Autodesk Fusion 360 part; units mm, degrees
note: some values were not read from the file. Set by a fixed rule: which sketch regions a step uses.
(part 16 of 59)
  spline S89 degree 5 poles (30.8773, 9.745) (30.8749, 9.7461) (30.87, 9.7485) (30.8627, 9.752) (30.853, 9.7566) (30.8408, 9.7624) (30.8287, 9.7681) (30.8165, 9.7738) (30.8044, 9.7795) (30.7924, 9.7851) (30.7803, 9.7908) (30.7683, 9.7964) (30.7563, 9.8019) (30.7443, 9.8075) (30.7323, 9.813) (30.7204, 9.8185) (30.7085, 9.8239) (30.6966, 9.8293) (30.6847, 9.8347) (30.6728, 9.8401) (30.661, 9.8455) (30.6492, 9.8508) (30.6374, 9.8561) (30.6256, 9.8613) (30.6139, 9.8665) (30.6022, 9.8717) (30.5905, 9.8769) (30.5788, 9.8821) (30.5672, 9.8872) (30.5555, 9.8923) (30.5439, 9.8973) (30.5324, 9.9023) (30.5208, 9.9073) (30.5093, 9.9123) (30.4978, 9.9173) (30.4863, 9.9222) (30.4749, 9.9271) (30.4634, 9.9319) (30.452, 9.9368) (30.4407, 9.9416) (30.4293, 9.9463) (30.418, 9.9511) (30.4067, 9.9558) (30.3954, 9.9605) (30.3841, 9.9652) (30.3729, 9.9698) (30.3617, 9.9744) (30.3506, 9.979) (30.3394, 9.9835) (30.3283, 9.9881) (30.3172, 9.9926) (30.3061, 9.997) (30.2951, 10.0015) (30.2841, 10.0059) (30.2731, 10.0103) (30.2621, 10.0146) (30.2512, 10.019) (30.2403, 10.0233) (30.2294, 10.0275) (30.2186, 10.0318) (30.2078, 10.036) (30.197, 10.0402) (30.1862, 10.0443) (30.1755, 10.0485) (30.1648, 10.0526) (30.1541, 10.0567) (30.1435, 10.0607) (30.1329, 10.0647) (30.1223, 10.0687) (30.1118, 10.0727) (30.1012, 10.0766) (30.0907, 10.0806) (30.0803, 10.0844) (30.0699, 10.0883) (30.0595, 10.0921) (30.0491, 10.0959) (30.0388, 10.0997) (30.0284, 10.1035) (30.0182, 10.1072) (30.0079, 10.1109) (29.9977, 10.1145) (29.9875, 10.1182) (29.9774, 10.1218) (29.9673, 10.1254) (29.9572, 10.1289) (29.9471, 10.1325) (29.9371, 10.136) (29.9271, 10.1394) (29.9172, 10.1429) (29.9073, 10.1463) (29.8974, 10.1497) (29.8875, 10.1531) (29.8777, 10.1564) (29.868, 10.1597) (29.8582, 10.163) (29.8485, 10.1663) (29.8388, 10.1695) (29.8292, 10.1727) (29.8196, 10.1759) (29.81, 10.179) (29.8005, 10.1822) (29.791, 10.1853) (29.7815, 10.1883) (29.7721, 10.1914) (29.7627, 10.1944) (29.7534, 10.1974) (29.7441, 10.2004) (29.7348, 10.2033) (29.7255, 10.2062) (29.7163, 10.2091) (29.7072, 10.212) (29.6981, 10.2148) (29.689, 10.2176) (29.6799, 10.2204) (29.6709, 10.2231) (29.6619, 10.2259) (29.653, 10.2286) (29.6441, 10.2312) (29.6353, 10.2339) (29.6265, 10.2365) (29.6177, 10.2391) (29.609, 10.2417) (29.6003, 10.2442) (29.5917, 10.2467) (29.583, 10.2492) (29.5745, 10.2517) (29.566, 10.2542) (29.5575, 10.2566) (29.5491, 10.259) (29.5407, 10.2613) (29.5323, 10.2637) (29.524, 10.266) (29.5158, 10.2683) (29.5075, 10.2705) (29.4994, 10.2728) (29.4912, 10.275) (29.4832, 10.2772) (29.4751, 10.2793) (29.4671, 10.2815) (29.4592, 10.2836) (29.4513, 10.2857) (29.4434, 10.2877) (29.4356, 10.2898) (29.4279, 10.2918) (29.4202, 10.2938) (29.4125, 10.2957) (29.4049, 10.2977) (29.3973, 10.2996) (29.3898, 10.3015) (29.3823, 10.3033) (29.3749, 10.3052) (29.3675, 10.307) (29.3602, 10.3088) (29.3529, 10.3105) (29.3457, 10.3123) (29.3386, 10.314) (29.3314, 10.3157) (29.3244, 10.3173) (29.3174, 10.319) (29.3104, 10.3206) (29.3035, 10.3222) (29.2967, 10.3238) (29.2899, 10.3253) (29.2831, 10.3269) (29.2764, 10.3284) (29.2698, 10.3298) (29.2632, 10.3313) (29.2567, 10.3327) (29.2502, 10.3341) (29.2438, 10.3355) (29.2374, 10.3369) (29.2311, 10.3382) (29.2249, 10.3395) (29.2187, 10.3408) (29.2126, 10.3421) (29.2065, 10.3433) (29.2005, 10.3446) (29.1946, 10.3458) (29.1887, 10.347) (29.1829, 10.3481) (29.1771, 10.3493) (29.1714, 10.3504) (29.1658, 10.3515) (29.1602, 10.3525) (29.1547, 10.3536) (29.1493, 10.3546) (29.1439, 10.3556) (29.1386, 10.3566) (29.1334, 10.3576) (29.1282, 10.3585) (29.1231, 10.3594) (29.118, 10.3603) (29.1131, 10.3612) (29.1081, 10.362) (29.1033, 10.3629) (29.0985, 10.3637) (29.0938, 10.3645) (29.0892, 10.3653) (29.0847, 10.366) (29.0802, 10.3668) (29.0758, 10.3675) (29.0714, 10.3682) (29.0672, 10.3688) (29.063, 10.3695) (29.0589, 10.3701) (29.0549, 10.3708) (29.0509, 10.3714) (29.047, 10.3719) (29.0432, 10.3725) (29.0395, 10.373) (29.0359, 10.3736) (29.0323, 10.3741) (29.0289, 10.3746) (29.0255, 10.375) (29.0222, 10.3755) (29.0189, 10.3759) (29.0158, 10.3763) (29.0128, 10.3767) (29.0098, 10.3771) (29.0069, 10.3775) (29.0041, 10.3778) (29.0015, 10.3781) (28.9989, 10.3785) (28.9963, 10.3788) (28.9939, 10.379) (28.9916, 10.3793) (28.9894, 10.3796) (28.9873, 10.3798) (28.9852, 10.38) (28.9833, 10.3802) (28.9815, 10.3804) (28.9798, 10.3806) (28.9781, 10.3808) (28.9766, 10.3809) (28.9752, 10.3811) (28.9739, 10.3812) (28.9727, 10.3813) (28.9716, 10.3814) (28.9706, 10.3815) (28.9698, 10.3816) (28.969, 10.3816) (28.9685, 10.3817) (28.9682, 10.3817) (28.968, 10.3817) (28.9679, 10.3817) knots -1 -1 -1 -1 -1 -1 -0.99583333 -0.99166667 -0.9875 -0.98333333 -0.97916667 -0.975 -0.97083333 -0.96666667 -0.9625 -0.95833333 -0.95416667 -0.95 -0.94583333 -0.94166667 -0.9375 -0.93333333 -0.92916667 -0.925 -0.92083333 -0.91666667 -0.9125 -0.90833333 -0.90416667 -0.9 -0.89583333 -0.89166667 -0.8875 -0.88333333 -0.87916667 -0.875 -0.87083333 -0.86666667 -0.8625 -0.85833333 -0.85416667 -0.85 -0.84583333 -0.84166667 -0.8375 -0.83333333 -0.82916667 -0.825 -0.82083333 -0.81666667 -0.8125 -0.80833333 -0.80416667 -0.8 -0.79583333 -0.79166667 -0.7875 -0.78333333 -0.77916667 -0.775 -0.77083333 -0.76666667 -0.7625 -0.75833333 -0.75416667 -0.75 -0.74583333 -0.74166667 -0.7375 -0.73333333 -0.72916667 -0.725 -0.72083333 -0.71666667 -0.7125 -0.70833333 -0.70416667 -0.7 -0.69583333 -0.69166667 -0.6875 -0.68333333 -0.67916667 -0.675 -0.67083333 -0.66666667 -0.6625 -0.65833333 -0.65416667 -0.65 -0.64583333 -0.64166667 -0.6375 -0.63333333 -0.62916667 -0.625 -0.62083333 -0.61666667 -0.6125 -0.60833333 -0.60416667 -0.6 -0.59583333 -0.59166667 -0.5875 -0.58333333 -0.57916667 -0.575 -0.57083333 -0.56666667 -0.5625 -0.55833333 -0.55416667 -0.55 -0.54583333 -0.54166667 -0.5375 -0.53333333 -0.52916667 -0.525 -0.52083333 -0.51666667 -0.5125 -0.50833333 -0.50416667 -0.5 -0.49583333 -0.49166667 -0.4875 -0.48333333 -0.47916667 -0.475 -0.47083333 -0.46666667 -0.4625 -0.45833333 -0.45416667 -0.45 -0.44583333 -0.44166667 -0.4375 -0.43333333 -0.42916667 -0.425 -0.42083333 -0.41666667 -0.4125 -0.40833333 -0.40416667 -0.4 -0.39583333 -0.39166667 -0.3875 -0.38333333 -0.37916667 -0.375 -0.37083333 -0.36666667 -0.3625 -0.35833333 -0.35416667 -0.35 -0.34583333 -0.34166667 -0.3375 -0.33333333 -0.32916667 -0.325 -0.32083333 -0.31666667 -0.3125 -0.30833333 -0.30416667 -0.3 -0.29583333 -0.29166667 -0.2875 -0.28333333 -0.27916667 -0.275 -0.27083333 -0.26666667 -0.2625 -0.25833333 -0.25416667 -0.25 -0.24583333 -0.24166667 -0.2375 -0.23333333 -0.22916667 -0.225 -0.22083333 -0.21666667 -0.2125 -0.20833333 -0.20416667 -0.2 -0.19583333 -0.19166667 -0.1875 -0.18333333 -0.17916667 -0.175 -0.17083333 -0.16666667 -0.1625 -0.15833333 -0.15416667 -0.15 -0.14583333 -0.14166667 -0.1375 -0.13333333 -0.12916667 -0.125 -0.12083333 -0.11666667 -0.1125 -0.10833333 -0.10416667 -0.1 -0.09583333 -0.09166667 -0.0875 -0.08333333 -0.07916667 -0.075 -0.07083333 -0.06666667 -0.0625 -0.05833333 -0.05416667 -0.05 -0.04583333 -0.04166667 -0.0375 -0.03333333 -0.02916667 -0.025 -0.02083333 -0.01666667 -0.0125 -0.00833333 -0.00416667 0 0 0 0 0 0
  spline S90 degree 5 poles (27.3251, 2.6528) (27.3252, 2.6528) (27.3254, 2.6527) (27.3257, 2.6526) (27.3262, 2.6525) (27.3269, 2.6522) (27.3277, 2.6519) (27.3286, 2.6516) (27.3296, 2.6513) (27.3308, 2.6509) (27.332, 2.6505) (27.3334, 2.65) (27.3348, 2.6495) (27.3364, 2.649) (27.338, 2.6485) (27.3398, 2.6479) (27.3416, 2.6473) (27.3435, 2.6467) (27.3456, 2.6461) (27.3477, 2.6454) (27.3499, 2.6447) (27.3523, 2.644) (27.3547, 2.6432) (27.3572, 2.6425) (27.3598, 2.6417) (27.3625, 2.6409) (27.3652, 2.64) (27.3681, 2.6392) (27.371, 2.6383) (27.3741, 2.6374) (27.3772, 2.6365) (27.3804, 2.6355) (27.3837, 2.6346) (27.387, 2.6336) (27.3905, 2.6326) (27.394, 2.6316) (27.3976, 2.6306) (27.4013, 2.6296) (27.4051, 2.6285) (27.409, 2.6275) (27.4129, 2.6264) (27.4169, 2.6253) (27.421, 2.6242) (27.4252, 2.6231) (27.4294, 2.622) (27.4337, 2.6208) (27.4381, 2.6197) (27.4426, 2.6185) (27.4471, 2.6173) (27.4517, 2.6162) (27.4564, 2.615) (27.4612, 2.6138) (27.466, 2.6126) (27.4709, 2.6113) (27.4759, 2.6101) (27.481, 2.6089) (27.4861, 2.6076) (27.4912, 2.6064) (27.4965, 2.6051) (27.5018, 2.6038) (27.5072, 2.6026) (27.5127, 2.6013) (27.5182, 2.6) (27.5238, 2.5987) (27.5294, 2.5974) (27.5352, 2.5961) (27.5409, 2.5948) (27.5468, 2.5935) (27.5527, 2.5921) (27.5587, 2.5908) (27.5647, 2.5895) (27.5709, 2.5882) (27.577, 2.5868) (27.5833, 2.5855) (27.5896, 2.5842) (27.5959, 2.5828) (27.6023, 2.5815) (27.6088, 2.5801) (27.6154, 2.5788) (27.622, 2.5775) (27.6286, 2.5761) (27.6353, 2.5748) (27.6421, 2.5734) (27.649, 2.5721) (27.6559, 2.5707) (27.6628, 2.5694) (27.6698, 2.568) (27.6769, 2.5667) (27.6841, 2.5653) (27.6912, 2.564) (27.6985, 2.5626) (27.7058, 2.5613) (27.7132, 2.5599) (27.7206, 2.5586) (27.728, 2.5572) (27.7356, 2.5559) (27.7431, 2.5546) (27.7508, 2.5532) (27.7585, 2.5519) (27.7662, 2.5506) (27.774, 2.5492) (27.7819, 2.5479) (27.7898, 2.5466) (27.7977, 2.5453) (27.8057, 2.544) (27.8138, 2.5427) (27.8219, 2.5414) (27.8301, 2.5401) (27.8383, 2.5388) (27.8466, 2.5375) (27.8549, 2.5362) (27.8633, 2.5349) (27.8717, 2.5336) (27.8802, 2.5324) (27.8887, 2.5311) (27.8973, 2.5299) (27.9059, 2.5286) (27.9146, 2.5274) (27.9233, 2.5261) (27.9321, 2.5249) (27.9409, 2.5237) (27.9498, 2.5224) (27.9587, 2.5212) (27.9677, 2.52) (27.9767, 2.5188) (27.9858, 2.5176) (27.9949, 2.5164) (28.004, 2.5153) (28.0133, 2.5141) (28.0225, 2.5129) (28.0318, 2.5118) (28.0412, 2.5106) (28.0506, 2.5095) (28.06, 2.5084) (28.0695, 2.5072) (28.079, 2.5061) (28.0886, 2.505) (28.0982, 2.5039) (28.1079, 2.5028) (28.1176, 2.5017) (28.1274, 2.5007) (28.1372, 2.4996) (28.147, 2.4986) (28.1569, 2.4975) (28.1668, 2.4965) (28.1768, 2.4955) (28.1868, 2.4945) (28.1969, 2.4935) (28.207, 2.4925) (28.2172, 2.4915) (28.2274, 2.4905) (28.2376, 2.4896) (28.2479, 2.4886) (28.2582, 2.4877) (28.2686, 2.4867) (28.279, 2.4858) (28.2894, 2.4849) (28.2999, 2.484) (28.3105, 2.4831) (28.321, 2.4823) (28.3317, 2.4814) (28.3423, 2.4805) (28.353, 2.4797) (28.3638, 2.4789) (28.3745, 2.4781) (28.3854, 2.4773) (28.3962, 2.4765) (28.4071, 2.4757) (28.4181, 2.4749) (28.429, 2.4742) (28.44, 2.4734) (28.4511, 2.4727) (28.4622, 2.472) (28.4733, 2.4713) (28.4845, 2.4706) (28.4957, 2.4699) (28.507, 2.4692) (28.5183, 2.4686) (28.5296, 2.4679) (28.541, 2.4673) (28.5524, 2.4667) (28.5638, 2.4661) (28.5753, 2.4655) (28.5868, 2.4649) (28.5984, 2.4644) (28.61, 2.4638) (28.6216, 2.4633) (28.6333, 2.4628) (28.645, 2.4623) (28.6567, 2.4618) (28.6685, 2.4613) (28.6803, 2.4608) (28.6922, 2.4604) (28.7041, 2.46) (28.716, 2.4595) (28.728, 2.4591) (28.74, 2.4588) (28.752, 2.4584) (28.7641, 2.458) (28.7762, 2.4577) (28.7883, 2.4573) (28.8005, 2.457) (28.8127, 2.4567) (28.8249, 2.4564) (28.8372, 2.4562) (28.8495, 2.4559) (28.8619, 2.4557) (28.8743, 2.4555) (28.8867, 2.4552) (28.8991, 2.4551) (28.9116, 2.4549) (28.9241, 2.4547) (28.9367, 2.4546) (28.9493, 2.4544) (28.9619, 2.4543) (28.9745, 2.4542) (28.9872, 2.4542) (29, 2.4541) (29.0127, 2.454) (29.0255, 2.454) (29.0383, 2.454) (29.0512, 2.454) (29.0641, 2.454) (29.077, 2.454) (29.0899, 2.4541) (29.1029, 2.4542) (29.1159, 2.4542) (29.129, 2.4543) (29.142, 2.4545) (29.1551, 2.4546) (29.1683, 2.4547) (29.1815, 2.4549) (29.1947, 2.4551) (29.2079, 2.4553) (29.2212, 2.4555) (29.2345, 2.4558) (29.2478, 2.456) (29.2612, 2.4563) (29.2745, 2.4566) (29.288, 2.4569) (29.3014, 2.4572) (29.3122, 2.4575) (29.3203, 2.4577) (29.3257, 2.4578) (29.3284, 2.4579) knots 0 0 0 0 0 0 0.00416667 0.00833333 0.0125 0.01666667 0.02083333 0.025 0.02916667 0.03333333 0.0375 0.04166667 0.04583333 0.05 0.05416667 0.05833333 0.0625 0.06666667 0.07083333 0.075 0.07916667 0.08333333 0.0875 0.09166667 0.09583333 0.1 0.10416667 0.10833333 0.1125 0.11666667 0.12083333 0.125 0.12916667 0.13333333 0.1375 0.14166667 0.14583333 0.15 0.15416667 0.15833333 0.1625 0.16666667 0.17083333 0.175 0.17916667 0.18333333 0.1875 0.19166667 0.19583333 0.2 0.20416667 0.20833333 0.2125 0.21666667 0.22083333 0.225 0.22916667 0.23333333 0.2375 0.24166667 0.24583333 0.25 0.25416667 0.25833333 0.2625 0.26666667 0.27083333 0.275 0.27916667 0.28333333 0.2875 0.29166667 0.29583333 0.3 0.30416667 0.30833333 0.3125 0.31666667 0.32083333 0.325 0.32916667 0.33333333 0.3375 0.34166667 0.34583333 0.35 0.35416667 0.35833333 0.3625 0.36666667 0.37083333 0.375 0.37916667 0.38333333 0.3875 0.39166667 0.39583333 0.4 0.40416667 0.40833333 0.4125 0.41666667 0.42083333 0.425 0.42916667 0.43333333 0.4375 0.44166667 0.44583333 0.45 0.45416667 0.45833333 0.4625 0.46666667 0.47083333 0.475 0.47916667 0.48333333 0.4875 0.49166667 0.49583333 0.5 0.50416667 0.50833333 0.5125 0.51666667 0.52083333 0.525 0.52916667 0.53333333 0.5375 0.54166667 0.54583333 0.55 0.55416667 0.55833333 0.5625 0.56666667 0.57083333 0.575 0.57916667 0.58333333 0.5875 0.59166667 0.59583333 0.6 0.60416667 0.60833333 0.6125 0.61666667 0.62083333 0.625 0.62916667 0.63333333 0.6375 0.64166667 0.64583333 0.65 0.65416667 0.65833333 0.6625 0.66666667 0.67083333 0.675 0.67916667 0.68333333 0.6875 0.69166667 0.69583333 0.7 0.70416667 0.70833333 0.7125 0.71666667 0.72083333 0.725 0.72916667 0.73333333 0.7375 0.74166667 0.74583333 0.75 0.75416667 0.75833333 0.7625 0.76666667 0.77083333 0.775 0.77916667 0.78333333 0.7875 0.79166667 0.79583333 0.8 0.80416667 0.80833333 0.8125 0.81666667 0.82083333 0.825 0.82916667 0.83333333 0.8375 0.84166667 0.84583333 0.85 0.85416667 0.85833333 0.8625 0.86666667 0.87083333 0.875 0.87916667 0.88333333 0.8875 0.89166667 0.89583333 0.9 0.90416667 0.90833333 0.9125 0.91666667 0.92083333 0.925 0.92916667 0.93333333 0.9375 0.94166667 0.94583333 0.95 0.95416667 0.95833333 0.9625 0.96666667 0.97083333 0.975 0.97916667 0.98333333 0.9875 0.99166667 0.99583333 1 1 1 1 1 1
  arc A96 (5.0824, 40.7972) -> (3.9106, 40.9828) centre (0, 12.5) ccw
  arc A97 (13.0527, 40.6181) -> (12.1618, 41.0147) centre (0, 12.5) ccw
  arc A98 (10.0421, 41.8284) -> (9.1146, 42.1298) centre (0, 12.5) ccw
  line L180 (12.6491, 38.6453) -> (12.6495, 38.6461)
  line L181 (12.5209, 38.3803) -> (12.6491, 38.6453)
  line L182 (13.7175, 38.1019) -> (13.7171, 38.1012)
  line L183 (10.9662, 39.3955) -> (10.9659, 39.3948)
  line L184 (29.0307, 13.4213) -> (29.0298, 13.4213)
  line L185 (8.0948, 40.3945) -> (8.0945, 40.3937)
  line L186 (9.7471, 39.5473) -> (9.8469, 39.8243)
  line L187 (-3.9507, -16.2745) -> (-3.9508, -16.2753)
  line L188 (29.0298, 13.4213) -> (28.7355, 13.4119)
  line L189 (10.9659, 39.3948) -> (10.8547, 39.1221)
  line L190 (8.0945, 40.3937) -> (8.0125, 40.1109)
  spline S91 degree 5 poles (30.4202, 6.5325) (30.4179, 6.5339) (30.4133, 6.5367) (30.4064, 6.541) (30.3972, 6.5466) (30.3857, 6.5536) (30.3742, 6.5606) (30.3628, 6.5675) (30.3513, 6.5745) (30.3399, 6.5813) (30.3285, 6.5882) (30.3171, 6.595) (30.3058, 6.6018) (30.2944, 6.6086) (30.2831, 6.6153) (30.2718, 6.622) (30.2605, 6.6287) (30.2492, 6.6353) (30.238, 6.6419) (30.2268, 6.6485) (30.2156, 6.6551) (30.2044, 6.6616) (30.1932, 6.6681) (30.1821, 6.6745) (30.1709, 6.6809) (30.1598, 6.6873) (30.1487, 6.6937) (30.1377, 6.7) (30.1266, 6.7063) (30.1156, 6.7126) (30.1046, 6.7189) (30.0936, 6.7251) (30.0826, 6.7312) (30.0717, 6.7374) (30.0608, 6.7435) (30.0499, 6.7496) (30.039, 6.7557) (30.0281, 6.7617) (30.0173, 6.7677) (30.0065, 6.7737) (29.9957, 6.7796) (29.9849, 6.7855) (29.9742, 6.7914) (29.9634, 6.7972) (29.9527, 6.803) (29.9421, 6.8088) (29.9314, 6.8146) (29.9208, 6.8203) (29.9102, 6.826) (29.8996, 6.8317) (29.889, 6.8373) (29.8785, 6.8429) (29.868, 6.8485) (29.8575, 6.854) (29.847, 6.8595) (29.8366, 6.865) (29.8262, 6.8704) (29.8158, 6.8758) (29.8054, 6.8812) (29.7951, 6.8866) (29.7847, 6.8919) (29.7745, 6.8972) (29.7642, 6.9025) (29.754, 6.9077) (29.7437, 6.9129) (29.7336, 6.9181) (29.7234, 6.9232) (29.7133, 6.9283) (29.7032, 6.9334) (29.6931, 6.9385) (29.683, 6.9435) (29.673, 6.9485) (29.663, 6.9534) (29.653, 6.9584) (29.6431, 6.9633) (29.6332, 6.9681) (29.6233, 6.973) (29.6134, 6.9778) (29.6036, 6.9825) (29.5938, 6.9873) (29.584, 6.992) (29.5743, 6.9967) (29.5646, 7.0013) (29.5549, 7.006) (29.5452, 7.0105) (29.5356, 7.0151) (29.526, 7.0196) (29.5165, 7.0241) (29.5069, 7.0286) (29.4974, 7.033) (29.4879, 7.0375) (29.4785, 7.0418) (29.4691, 7.0462) (29.4597, 7.0505) (29.4504, 7.0548) (29.441, 7.059) (29.4318, 7.0633) (29.4225, 7.0675) (29.4133, 7.0716) (29.4041, 7.0758) (29.395, 7.0799) (29.3858, 7.0839) (29.3767, 7.088) (29.3677, 7.092) (29.3587, 7.096) (29.3497, 7.0999) (29.3407, 7.1039) (29.3318, 7.1078) (29.3229, 7.1116) (29.3141, 7.1154) (29.3053, 7.1193) (29.2965, 7.123) (29.2878, 7.1268) (29.279, 7.1305) (29.2704, 7.1342) (29.2617, 7.1378) (29.2531, 7.1414) (29.2446, 7.145) (29.2361, 7.1486) (29.2276, 7.1521) (29.2191, 7.1556) (29.2107, 7.1591) (29.2023, 7.1625) (29.194, 7.1659) (29.1857, 7.1693) (29.1775, 7.1727) (29.1692, 7.176) (29.1611, 7.1793) (29.1529, 7.1825) (29.1448, 7.1857) (29.1368, 7.1889) (29.1288, 7.1921) (29.1208, 7.1953) (29.1129, 7.1984) (29.105, 7.2014) (29.0971, 7.2045) (29.0893, 7.2075) (29.0815, 7.2105) (29.0738, 7.2135) (29.0661, 7.2164) (29.0585, 7.2193) (29.0509, 7.2222) (29.0433, 7.225) (29.0358, 7.2278) (29.0284, 7.2306) (29.021, 7.2334) (29.0136, 7.2361) (29.0063, 7.2388) (28.999, 7.2414) (28.9918, 7.2441) (28.9846, 7.2467) (28.9774, 7.2492) (28.9703, 7.2518) (28.9633, 7.2543) (28.9563, 7.2568) (28.9493, 7.2592) (28.9424, 7.2617) (28.9356, 7.2641) (28.9288, 7.2664) (28.922, 7.2688) (28.9153, 7.2711) (28.9087, 7.2734) (28.9021, 7.2756) (28.8955, 7.2778) (28.889, 7.28) (28.8826, 7.2822) (28.8762, 7.2843) (28.8699, 7.2864) (28.8636, 7.2885) (28.8573, 7.2906) (28.8512, 7.2926) (28.8451, 7.2946) (28.839, 7.2965) (28.833, 7.2985) (28.827, 7.3004) (28.8211, 7.3022) (28.8153, 7.3041) (28.8095, 7.3059) (28.8038, 7.3077) (28.7981, 7.3095) (28.7925, 7.3112) (28.7869, 7.3129) (28.7815, 7.3146) (28.776, 7.3162) (28.7707, 7.3178) (28.7654, 7.3194) (28.7601, 7.321) (28.7549, 7.3225) (28.7498, 7.324) (28.7448, 7.3255) (28.7398, 7.327) (28.7349, 7.3284) (28.73, 7.3298) (28.7252, 7.3311) (28.7205, 7.3325) (28.7158, 7.3338) (28.7112, 7.3351) (28.7067, 7.3363) (28.7023, 7.3375) (28.6979, 7.3387) (28.6936, 7.3399) (28.6893, 7.3411) (28.6852, 7.3422) (28.6811, 7.3433) (28.6771, 7.3443) (28.6731, 7.3454) (28.6693, 7.3464) (28.6655, 7.3473) (28.6617, 7.3483) (28.6581, 7.3492) (28.6545, 7.3501) (28.6511, 7.351) (28.6477, 7.3519) (28.6443, 7.3527) (28.6411, 7.3535) (28.6379, 7.3542) (28.6349, 7.355) (28.6319, 7.3557) (28.629, 7.3564) (28.6262, 7.357) (28.6234, 7.3577) (28.6208, 7.3583) (28.6182, 7.3589) (28.6158, 7.3594) (28.6134, 7.36) (28.6111, 7.3605) (28.6089, 7.361) (28.6069, 7.3614) (28.6049, 7.3619) (28.603, 7.3623) (28.6012, 7.3626) (28.5995, 7.363) (28.5979, 7.3633) (28.5964, 7.3637) (28.595, 7.3639) (28.5937, 7.3642) (28.5925, 7.3644) (28.5915, 7.3646) (28.5905, 7.3648) (28.5896, 7.365) (28.5889, 7.3651) (28.5884, 7.3652) (28.5881, 7.3653) (28.5879, 7.3653) (28.5878, 7.3654) knots -1 -1 -1 -1 -1 -1 -0.99583333 -0.99166667 -0.9875 -0.98333333 -0.97916667 -0.975 -0.97083333 -0.96666667 -0.9625 -0.95833333 -0.95416667 -0.95 -0.94583333 -0.94166667 -0.9375 -0.93333333 -0.92916667 -0.925 -0.92083333 -0.91666667 -0.9125 -0.90833333 -0.90416667 -0.9 -0.89583333 -0.89166667 -0.8875 -0.88333333 -0.87916667 -0.875 -0.87083333 -0.86666667 -0.8625 -0.85833333 -0.85416667 -0.85 -0.84583333 -0.84166667 -0.8375 -0.83333333 -0.82916667 -0.825 -0.82083333 -0.81666667 -0.8125 -0.80833333 -0.80416667 -0.8 -0.79583333 -0.79166667 -0.7875 -0.78333333 -0.77916667 -0.775 -0.77083333 -0.76666667 -0.7625 -0.75833333 -0.75416667 -0.75 -0.74583333 -0.74166667 -0.7375 -0.73333333 -0.72916667 -0.725 -0.72083333 -0.71666667 -0.7125 -0.70833333 -0.70416667 -0.7 -0.69583333 -0.69166667 -0.6875 -0.68333333 -0.67916667 -0.675 -0.67083333 -0.66666667 -0.6625 -0.65833333 -0.65416667 -0.65 -0.64583333 -0.64166667 -0.6375 -0.63333333 -0.62916667 -0.625 -0.62083333 -0.61666667 -0.6125 -0.60833333 -0.60416667 -0.6 -0.59583333 -0.59166667 -0.5875 -0.58333333 -0.57916667 -0.575 -0.57083333 -0.56666667 -0.5625 -0.55833333 -0.55416667 -0.55 -0.54583333 -0.54166667 -0.5375 -0.53333333 -0.52916667 -0.525 -0.52083333 -0.51666667 -0.5125 -0.50833333 -0.50416667 -0.5 -0.49583333 -0.49166667 -0.4875 -0.48333333 -0.47916667 -0.475 -0.47083333 -0.46666667 -0.4625 -0.45833333 -0.45416667 -0.45 -0.44583333 -0.44166667 -0.4375 -0.43333333 -0.42916667 -0.425 -0.42083333 -0.41666667 -0.4125 -0.40833333 -0.40416667 -0.4 -0.39583333 -0.39166667 -0.3875 -0.38333333 -0.37916667 -0.375 -0.37083333 -0.36666667 -0.3625 -0.35833333 -0.35416667 -0.35 -0.34583333 -0.34166667 -0.3375 -0.33333333 -0.32916667 -0.325 -0.32083333 -0.31666667 -0.3125 -0.30833333 -0.30416667 -0.3 -0.29583333 -0.29166667 -0.2875 -0.28333333 -0.27916667 -0.275 -0.27083333 -0.26666667 -0.2625 -0.25833333 -0.25416667 -0.25 -0.24583333 -0.24166667 -0.2375 -0.23333333 -0.22916667 -0.225 -0.22083333 -0.21666667 -0.2125 -0.20833333 -0.20416667 -0.2 -0.19583333 -0.19166667 -0.1875 -0.18333333 -0.17916667 -0.175 -0.17083333 -0.16666667 -0.1625 -0.15833333 -0.15416667 -0.15 -0.14583333 -0.14166667 -0.1375 -0.13333333 -0.12916667 -0.125 -0.12083333 -0.11666667 -0.1125 -0.10833333 -0.10416667 -0.1 -0.09583333 -0.09166667 -0.0875 -0.08333333 -0.07916667 -0.075 -0.07083333 -0.06666667 -0.0625 -0.05833333 -0.05416667 -0.05 -0.04583333 -0.04166667 -0.0375 -0.03333333 -0.02916667 -0.025 -0.02083333 -0.01666667 -0.0125 -0.00833333 -0.00416667 0 0 0 0 0 0
  arc A99 (13.578, 37.8417) -> (12.5209, 38.3803) centre (0, 12.5) ccw
  line L191 (13.7171, 38.1012) -> (13.578, 37.8417)
  line L192 (9.8469, 39.8243) -> (9.8472, 39.8251)
  line L193 (6.937, -15.7047) -> (6.9368, -15.7039)
  arc A100 (10.8547, 39.1221) -> (9.7471, 39.5473) centre (0, 12.5) ccw
  line L194 (-3.9106, -15.9828) -> (-3.9507, -16.2745)
  line L195 (6.9368, -15.7039) -> (6.8665, -15.418)
  line L196 (24.6799, -2.8128) -> (24.6806, -2.8132)
  line L197 (13.7171, -13.1012) -> (13.7175, -13.1019)
  arc A101 (23.7836, -3.6526) -> (24.4297, -2.6575) centre (0, 12.5) ccw
  line L198 (25.8803, -0.0209) -> (26.1453, -0.1491)
  line L199 (16.1526, -11.2836) -> (16.318, -11.5271)
  line L200 (27.3251, 22.3472) -> (27.3243, 22.3469)
  spline S92 degree 5 poles (15.0758, 39.5873) (15.0737, 39.5855) (15.0696, 39.582) (15.0635, 39.5767) (15.0553, 39.5697) (15.045, 39.561) (15.0349, 39.5522) (15.0247, 39.5435) (15.0146, 39.5347) (15.0045, 39.526) (14.9945, 39.5173) (14.9845, 39.5086) (14.9745, 39.4999) (14.9646, 39.4912) (14.9547, 39.4825) (14.9448, 39.4738) (14.935, 39.4651) (14.9252, 39.4565) (14.9154, 39.4478) (14.9057, 39.4392) (14.896, 39.4305) (14.8863, 39.4219) (14.8767, 39.4133) (14.8671, 39.4047) (14.8576, 39.3961) (14.8481, 39.3875) (14.8386, 39.3789) (14.8291, 39.3703) (14.8197, 39.3618) (14.8104, 39.3532) (14.801, 39.3447) (14.7917, 39.3361) (14.7824, 39.3276) (14.7732, 39.3191) (14.764, 39.3106) (14.7549, 39.3021) (14.7457, 39.2937) (14.7366, 39.2852) (14.7276, 39.2767) (14.7186, 39.2683) (14.7096, 39.2599) (14.7006, 39.2515) (14.6917, 39.2431) (14.6829, 39.2347) (14.674, 39.2263) (14.6652, 39.2179) (14.6565, 39.2096) (14.6477, 39.2012) (14.639, 39.1929) (14.6304, 39.1846) (14.6218, 39.1763) (14.6132, 39.168) (14.6046, 39.1597) (14.5961, 39.1514) (14.5877, 39.1432) (14.5792, 39.135) (14.5708, 39.1267) (14.5625, 39.1185) (14.5541, 39.1103) (14.5459, 39.1022) (14.5376, 39.094) (14.5294, 39.0858) (14.5212, 39.0777) (14.5131, 39.0696) (14.505, 39.0615) (14.4969, 39.0534) (14.4889, 39.0453) (14.4809, 39.0373) (14.4729, 39.0292) (14.465, 39.0212) (14.4571, 39.0132) (14.4493, 39.0052) (14.4415, 38.9972) (14.4337, 38.9893) (14.426, 38.9813) (14.4183, 38.9734) (14.4106, 38.9655) (14.403, 38.9576) (14.3954, 38.9497) (14.3879, 38.9419) (14.3804, 38.934) (14.3729, 38.9262) (14.3655, 38.9184) (14.3581, 38.9106) (14.3508, 38.9029) (14.3435, 38.8951) (14.3362, 38.8874) (14.3289, 38.8797) (14.3217, 38.872) (14.3146, 38.8643) (14.3075, 38.8567) (14.3004, 38.8491) (14.2933, 38.8414) (14.2863, 38.8339) (14.2794, 38.8263) (14.2724, 38.8188) (14.2656, 38.8112) (14.2587, 38.8037) (14.2519, 38.7962) (14.2451, 38.7888) (14.2384, 38.7813) (14.2317, 38.7739) (14.225, 38.7665) (14.2184, 38.7592) (14.2119, 38.7518) (14.2053, 38.7445) (14.1988, 38.7372) (14.1924, 38.7299) (14.1859, 38.7227) (14.1796, 38.7154) (14.1732, 38.7082) (14.1669, 38.701) (14.1607, 38.6939) (14.1544, 38.6868) (14.1483, 38.6796) (14.1421, 38.6726) (14.136, 38.6655) (14.13, 38.6585) (14.1239, 38.6515) (14.118, 38.6445) (14.112, 38.6375) (14.1061, 38.6306) (14.1003, 38.6237) (14.0945, 38.6168) (14.0887, 38.61) (14.0829, 38.6032) (14.0772, 38.5964) (14.0716, 38.5896) (14.066, 38.5829) (14.0604, 38.5762) (14.0549, 38.5695) (14.0494, 38.5629) (14.0439, 38.5563) (14.0385, 38.5497) (14.0332, 38.5431) (14.0278, 38.5366) (14.0225, 38.5301) (14.0173, 38.5236) (14.0121, 38.5172) (14.0069, 38.5108) (14.0018, 38.5044) (13.9967, 38.4981) (13.9917, 38.4918) (13.9867, 38.4855) (13.9818, 38.4793) (13.9769, 38.4731) (13.972, 38.4669) (13.9672, 38.4608) (13.9624, 38.4547) (13.9576, 38.4486) (13.9529, 38.4426) (13.9483, 38.4366) (13.9437, 38.4306) (13.9391, 38.4247) (13.9346, 38.4188) (13.9301, 38.413) (13.9257, 38.4072) (13.9213, 38.4014) (13.9169, 38.3957) (13.9126, 38.39) (13.9083, 38.3843) (13.9041, 38.3787) (13.8999, 38.3731) (13.8958, 38.3676) (13.8917, 38.3621) (13.8876, 38.3566) (13.8836, 38.3512) (13.8797, 38.3458) (13.8758, 38.3405) (13.8719, 38.3352) (13.8681, 38.3299) (13.8643, 38.3247) (13.8605, 38.3195) (13.8568, 38.3144) (13.8532, 38.3093) (13.8496, 38.3043) (13.846, 38.2993) (13.8425, 38.2944) (13.839, 38.2895) (13.8356, 38.2847) (13.8322, 38.2799) (13.8289, 38.2751) (13.8256, 38.2704) (13.8224, 38.2658) (13.8192, 38.2612) (13.816, 38.2566) (13.8129, 38.2521) (13.8098, 38.2476) (13.8068, 38.2432) (13.8039, 38.2389) (13.8009, 38.2346) (13.7981, 38.2304) (13.7952, 38.2262) (13.7925, 38.222) (13.7897, 38.218) (13.787, 38.2139) (13.7844, 38.21) (13.7818, 38.206) (13.7793, 38.2022) (13.7768, 38.1984) (13.7743, 38.1947) (13.7719, 38.191) (13.7696, 38.1874) (13.7673, 38.1838) (13.765, 38.1803) (13.7628, 38.1769) (13.7607, 38.1735) (13.7586, 38.1702) (13.7565, 38.167) (13.7545, 38.1638) (13.7526, 38.1607) (13.7506, 38.1577) (13.7488, 38.1547) (13.747, 38.1518) (13.7452, 38.1489) (13.7435, 38.1462) (13.7419, 38.1435) (13.7403, 38.1409) (13.7387, 38.1383) (13.7372, 38.1358) (13.7358, 38.1334) (13.7344, 38.1311) (13.733, 38.1289) (13.7317, 38.1267) (13.7305, 38.1246) (13.7293, 38.1226) (13.7282, 38.1207) (13.7271, 38.1188) (13.7261, 38.1171) (13.7251, 38.1154) (13.7242, 38.1138) (13.7233, 38.1123) (13.7225, 38.1109) (13.7217, 38.1096) (13.721, 38.1083) (13.7204, 38.1072) (13.7198, 38.1061) (13.7193, 38.1052) (13.7188, 38.1043) (13.7184, 38.1036) (13.718, 38.1029) (13.7178, 38.1025) (13.7176, 38.1022) (13.7175, 38.102) (13.7175, 38.1019) knots -1 -1 -1 -1 -1 -1 -0.99583333 -0.99166667 -0.9875 -0.98333333 -0.97916667 -0.975 -0.97083333 -0.96666667 -0.9625 -0.95833333 -0.95416667 -0.95 -0.94583333 -0.94166667 -0.9375 -0.93333333 -0.92916667 -0.925 -0.92083333 -0.91666667 -0.9125 -0.90833333 -0.90416667 -0.9 -0.89583333 -0.89166667 -0.8875 -0.88333333 -0.87916667 -0.875 -0.87083333 -0.86666667 -0.8625 -0.85833333 -0.85416667 -0.85 -0.84583333 -0.84166667 -0.8375 -0.83333333 -0.82916667 -0.825 -0.82083333 -0.81666667 -0.8125 -0.80833333 -0.80416667 -0.8 -0.79583333 -0.79166667 -0.7875 -0.78333333 -0.77916667 -0.775 -0.77083333 -0.76666667 -0.7625 -0.75833333 -0.75416667 -0.75 -0.74583333 -0.74166667 -0.7375 -0.73333333 -0.72916667 -0.725 -0.72083333 -0.71666667 -0.7125 -0.70833333 -0.70416667 -0.7 -0.69583333 -0.69166667 -0.6875 -0.68333333 -0.67916667 -0.675 -0.67083333 -0.66666667 -0.6625 -0.65833333 -0.65416667 -0.65 -0.64583333 -0.64166667 -0.6375 -0.63333333 -0.62916667 -0.625 -0.62083333 -0.61666667 -0.6125 -0.60833333 -0.60416667 -0.6 -0.59583333 -0.59166667 -0.5875 -0.58333333 -0.57916667 -0.575 -0.57083333 -0.56666667 -0.5625 -0.55833333 -0.55416667 -0.55 -0.54583333 -0.54166667 -0.5375 -0.53333333 -0.52916667 -0.525 -0.52083333 -0.51666667 -0.5125 -0.50833333 -0.50416667 -0.5 -0.49583333 -0.49166667 -0.4875 -0.48333333 -0.47916667 -0.475 -0.47083333 -0.46666667 -0.4625 -0.45833333 -0.45416667 -0.45 -0.44583333 -0.44166667 -0.4375 -0.43333333 -0.42916667 -0.425 -0.42083333 -0.41666667 -0.4125 -0.40833333 -0.40416667 -0.4 -0.39583333 -0.39166667 -0.3875 -0.38333333 -0.37916667 -0.375 -0.37083333 -0.36666667 -0.3625 -0.35833333 -0.35416667 -0.35 -0.34583333 -0.34166667 -0.3375 -0.33333333 -0.32916667 -0.325 -0.32083333 -0.31666667 -0.3125 -0.30833333 -0.30416667 -0.3 -0.29583333 -0.29166667 -0.2875 -0.28333333 -0.27916667 -0.275 -0.27083333 -0.26666667 -0.2625 -0.25833333 -0.25416667 -0.25 -0.24583333 -0.24166667 -0.2375 -0.23333333 -0.22916667 -0.225 -0.22083333 -0.21666667 -0.2125 -0.20833333 -0.20416667 -0.2 -0.19583333 -0.19166667 -0.1875 -0.18333333 -0.17916667 -0.175 -0.17083333 -0.16666667 -0.1625 -0.15833333 -0.15416667 -0.15 -0.14583333 -0.14166667 -0.1375 -0.13333333 -0.12916667 -0.125 -0.12083333 -0.11666667 -0.1125 -0.10833333 -0.10416667 -0.1 -0.09583333 -0.09166667 -0.0875 -0.08333333 -0.07916667 -0.075 -0.07083333 -0.06666667 -0.0625 -0.05833333 -0.05416667 -0.05 -0.04583333 -0.04166667 -0.0375 -0.03333333 -0.02916667 -0.025 -0.02083333 -0.01666667 -0.0125 -0.00833333 -0.00416667 0 0 0 0 0 0
  arc A102 (15.0758, -14.5873) -> (15.9204, -14.0997) centre (0, 12.5) ccw
  line L201 (24.4297, -2.6575) -> (24.6799, -2.8128)
  arc A103 (12.5209, -13.3803) -> (13.578, -12.8417) centre (0, 12.5) ccw
  line L202 (15.3128, -12.1799) -> (15.1575, -11.9297)
  spline S93 degree 5 poles (0.4876, -18.4962) (0.4885, -18.4936) (0.4903, -18.4885) (0.493, -18.4809) (0.4966, -18.4707) (0.5011, -18.458) (0.5055, -18.4453) (0.5099, -18.4327) (0.5143, -18.4201) (0.5187, -18.4075) (0.523, -18.3949) (0.5273, -18.3823) (0.5316, -18.3698) (0.5359, -18.3573) (0.5401, -18.3448) (0.5443, -18.3324) (0.5485, -18.32) (0.5526, -18.3076) (0.5568, -18.2952) (0.5609, -18.2828) (0.5649, -18.2705) (0.569, -18.2582) (0.573, -18.2459) (0.577, -18.2337) (0.581, -18.2215) (0.5849, -18.2093) (0.5889, -18.1971) (0.5927, -18.185) (0.5966, -18.1728) (0.6005, -18.1607) (0.6043, -18.1487) (0.6081, -18.1366) (0.6118, -18.1246) (0.6156, -18.1126) (0.6193, -18.1007) (0.623, -18.0888) (0.6267, -18.0769) (0.6303, -18.065) (0.6339, -18.0531) (0.6375, -18.0413) (0.6411, -18.0295) (0.6446, -18.0178) (0.6481, -18.006) (0.6516, -17.9943) (0.6551, -17.9827) (0.6585, -17.971) (0.6619, -17.9594) (0.6653, -17.9478) (0.6687, -17.9362) (0.672, -17.9247) (0.6753, -17.9132) (0.6786, -17.9017) (0.6819, -17.8903) (0.6851, -17.8789) (0.6883, -17.8675) (0.6915, -17.8562) (0.6947, -17.8448) (0.6978, -17.8336) (0.7009, -17.8223) (0.704, -17.8111) (0.7071, -17.7999) (0.7101, -17.7887) (0.7131, -17.7776) (0.7161, -17.7665) (0.7191, -17.7554) (0.722, -17.7444) (0.7249, -17.7334) (0.7278, -17.7224) (0.7307, -17.7114) (0.7335, -17.7005) (0.7364, -17.6897) (0.7391, -17.6788) (0.7419, -17.668) (0.7447, -17.6572) (0.7474, -17.6465) (0.7501, -17.6358) (0.7528, -17.6251) (0.7554, -17.6145) (0.758, -17.6038) (0.7606, -17.5933) (0.7632, -17.5827) (0.7658, -17.5722) (0.7683, -17.5618) (0.7708, -17.5513) (0.7733, -17.5409) (0.7758, -17.5306) (0.7782, -17.5202) (0.7806, -17.5099) (0.783, -17.4997) (0.7854, -17.4895) (0.7877, -17.4793) (0.79, -17.4691) (0.7923, -17.459) (0.7946, -17.449) (0.7969, -17.4389) (0.7991, -17.4289) (0.8013, -17.419) (0.8035, -17.409) (0.8056, -17.3992) (0.8078, -17.3893) (0.8099, -17.3795) (0.812, -17.3697) (0.814, -17.36) (0.8161, -17.3503) (0.8181, -17.3407) (0.8201, -17.3311) (0.8221, -17.3215) (0.824, -17.312) (0.8259, -17.3025) (0.8279, -17.293) (0.8297, -17.2836) (0.8316, -17.2742) (0.8334, -17.2649) (0.8353, -17.2556) (0.8371, -17.2464) (0.8388, -17.2372) (0.8406, -17.228) (0.8423, -17.2189) (0.844, -17.2098) (0.8457, -17.2008) (0.8474, -17.1918) (0.849, -17.1828) (0.8507, -17.1739) (0.8523, -17.1651) (0.8538, -17.1563) (0.8554, -17.1475) (0.8569, -17.1388) (0.8585, -17.1301) (0.86, -17.1214) (0.8614, -17.1128) (0.8629, -17.1043) (0.8643, -17.0958) (0.8657, -17.0873) (0.8671, -17.0789) (0.8685, -17.0706) (0.8698, -17.0623) (0.8712, -17.054) (0.8725, -17.0458) (0.8738, -17.0376) (0.875, -17.0295) (0.8763, -17.0214) (0.8775, -17.0134) (0.8787, -17.0054) (0.8799, -16.9975) (0.8811, -16.9896) (0.8822, -16.9818) (0.8834, -16.974) (0.8845, -16.9663) (0.8856, -16.9586) (0.8866, -16.951) (0.8877, -16.9434) (0.8887, -16.9359) (0.8897, -16.9284) (0.8907, -16.921) (0.8917, -16.9137) (0.8927, -16.9063) (0.8936, -16.8991) (0.8945, -16.8919) (0.8954, -16.8847) (0.8963, -16.8777) (0.8972, -16.8706) (0.898, -16.8636) (0.8989, -16.8567) (0.8997, -16.8498) (0.9005, -16.843) (0.9012, -16.8363) (0.902, -16.8296) (0.9027, -16.823) (0.9035, -16.8164) (0.9042, -16.8099) (0.9049, -16.8034) (0.9055, -16.797) (0.9062, -16.7906) (0.9068, -16.7844) (0.9075, -16.7781) (0.9081, -16.772) (0.9087, -16.7659) (0.9092, -16.7599) (0.9098, -16.7539) (0.9103, -16.748) (0.9109, -16.7421) (0.9114, -16.7363) (0.9119, -16.7306) (0.9124, -16.725) (0.9128, -16.7194) (0.9133, -16.7139) (0.9137, -16.7084) (0.9141, -16.703) (0.9146, -16.6977) (0.915, -16.6925) (0.9153, -16.6873) (0.9157, -16.6822) (0.9161, -16.6771) (0.9164, -16.6722) (0.9167, -16.6673) (0.917, -16.6624) (0.9173, -16.6577) (0.9176, -16.653) (0.9179, -16.6484) (0.9182, -16.6439) (0.9184, -16.6394) (0.9186, -16.635) (0.9189, -16.6307) (0.9191, -16.6265) (0.9193, -16.6223) (0.9195, -16.6183) (0.9197, -16.6143) (0.9198, -16.6103) (0.92, -16.6065) (0.9201, -16.6028) (0.9203, -16.5991) (0.9204, -16.5955) (0.9205, -16.592) (0.9206, -16.5886) (0.9208, -16.5852) (0.9208, -16.582) (0.9209, -16.5788) (0.921, -16.5758) (0.9211, -16.5728) (0.9211, -16.5699) (0.9212, -16.5671) (0.9212, -16.5644) (0.9213, -16.5618) (0.9213, -16.5592) (0.9214, -16.5568) (0.9214, -16.5545) (0.9214, -16.5522) (0.9214, -16.5501) (0.9214, -16.5481) (0.9214, -16.5461) (0.9214, -16.5443) (0.9214, -16.5425) (0.9214, -16.5409) (0.9214, -16.5394) (0.9214, -16.538) (0.9214, -16.5367) (0.9214, -16.5355) (0.9214, -16.5344) (0.9213, -16.5334) (0.9213, -16.5325) (0.9213, -16.5318) (0.9213, -16.5313) (0.9213, -16.5309) (0.9213, -16.5307) (0.9213, -16.5307) knots -1 -1 -1 -1 -1 -1 -0.99583333 -0.99166667 -0.9875 -0.98333333 -0.97916667 -0.975 -0.97083333 -0.96666667 -0.9625 -0.95833333 -0.95416667 -0.95 -0.94583333 -0.94166667 -0.9375 -0.93333333 -0.92916667 -0.925 -0.92083333 -0.91666667 -0.9125 -0.90833333 -0.90416667 -0.9 -0.89583333 -0.89166667 -0.8875 -0.88333333 -0.87916667 -0.875 -0.87083333 -0.86666667 -0.8625 -0.85833333 -0.85416667 -0.85 -0.84583333 -0.84166667 -0.8375 -0.83333333 -0.82916667 -0.825 -0.82083333 -0.81666667 -0.8125 -0.80833333 -0.80416667 -0.8 -0.79583333 -0.79166667 -0.7875 -0.78333333 -0.77916667 -0.775 -0.77083333 -0.76666667 -0.7625 -0.75833333 -0.75416667 -0.75 -0.74583333 -0.74166667 -0.7375 -0.73333333 -0.72916667 -0.725 -0.72083333 -0.71666667 -0.7125 -0.70833333 -0.70416667 -0.7 -0.69583333 -0.69166667 -0.6875 -0.68333333 -0.67916667 -0.675 -0.67083333 -0.66666667 -0.6625 -0.65833333 -0.65416667 -0.65 -0.64583333 -0.64166667 -0.6375 -0.63333333 -0.62916667 -0.625 -0.62083333 -0.61666667 -0.6125 -0.60833333 -0.60416667 -0.6 -0.59583333 -0.59166667 -0.5875 -0.58333333 -0.57916667 -0.575 -0.57083333 -0.56666667 -0.5625 -0.55833333 -0.55416667 -0.55 -0.54583333 -0.54166667 -0.5375 -0.53333333 -0.52916667 -0.525 -0.52083333 -0.51666667 -0.5125 -0.50833333 -0.50416667 -0.5 -0.49583333 -0.49166667 -0.4875 -0.48333333 -0.47916667 -0.475 -0.47083333 -0.46666667 -0.4625 -0.45833333 -0.45416667 -0.45 -0.44583333 -0.44166667 -0.4375 -0.43333333 -0.42916667 -0.425 -0.42083333 -0.41666667 -0.4125 -0.40833333 -0.40416667 -0.4 -0.39583333 -0.39166667 -0.3875 -0.38333333 -0.37916667 -0.375 -0.37083333 -0.36666667 -0.3625 -0.35833333 -0.35416667 -0.35 -0.34583333 -0.34166667 -0.3375 -0.33333333 -0.32916667 -0.325 -0.32083333 -0.31666667 -0.3125 -0.30833333 -0.30416667 -0.3 -0.29583333 -0.29166667 -0.2875 -0.28333333 -0.27916667 -0.275 -0.27083333 -0.26666667 -0.2625 -0.25833333 -0.25416667 -0.25 -0.24583333 -0.24166667 -0.2375 -0.23333333 -0.22916667 -0.225 -0.22083333 -0.21666667 -0.2125 -0.20833333 -0.20416667 -0.2 -0.19583333 -0.19166667 -0.1875 -0.18333333 -0.17916667 -0.175 -0.17083333 -0.16666667 -0.1625 -0.15833333 -0.15416667 -0.15 -0.14583333 -0.14166667 -0.1375 -0.13333333 -0.12916667 -0.125 -0.12083333 -0.11666667 -0.1125 -0.10833333 -0.10416667 -0.1 -0.09583333 -0.09166667 -0.0875 -0.08333333 -0.07916667 -0.075 -0.07083333 -0.06666667 -0.0625 -0.05833333 -0.05416667 -0.05 -0.04583333 -0.04166667 -0.0375 -0.03333333 -0.02916667 -0.025 -0.02083333 -0.01666667 -0.0125 -0.00833333 -0.00416667 0 0 0 0 0 0
  line L203 (25.6012, -1.2171) -> (25.3417, -1.078)
  line L204 (16.318, -11.5271) -> (16.3184, -11.5278)
  line L205 (27.3243, 22.3469) -> (27.0473, 22.2471)
  spline S94 degree 5 poles (-6.937, -15.7047) (-6.937, -15.7048) (-6.937, -15.705) (-6.9371, -15.7053) (-6.9372, -15.7058) (-6.9374, -15.7065) (-6.9376, -15.7074) (-6.9378, -15.7083) (-6.9381, -15.7094) (-6.9383, -15.7106) (-6.9386, -15.7118) (-6.9389, -15.7132) (-6.9392, -15.7147) (-6.9396, -15.7163) (-6.9399, -15.718) (-6.9403, -15.7198) (-6.9407, -15.7217) (-6.9411, -15.7237) (-6.9416, -15.7258) (-6.942, -15.728) (-6.9425, -15.7303) (-6.9429, -15.7327) (-6.9434, -15.7351) (-6.9439, -15.7377) (-6.9445, -15.7404) (-6.945, -15.7431) (-6.9455, -15.746) (-6.9461, -15.7489) (-6.9466, -15.7519) (-6.9472, -15.755) (-6.9478, -15.7582) (-6.9484, -15.7615) (-6.949, -15.7649) (-6.9496, -15.7683) (-6.9502, -15.7719) (-6.9508, -15.7755) (-6.9515, -15.7792) (-6.9521, -15.783) (-6.9528, -15.7868) (-6.9534, -15.7908) (-6.9541, -15.7948) (-6.9547, -15.7989) (-6.9554, -15.8031) (-6.9561, -15.8074) (-6.9568, -15.8117) (-6.9574, -15.8161) (-6.9581, -15.8206) (-6.9588, -15.8252) (-6.9595, -15.8298) (-6.9602, -15.8345) (-6.9609, -15.8393) (-6.9616, -15.8442) (-6.9623, -15.8491) (-6.963, -15.8541) (-6.9637, -15.8592) (-6.9644, -15.8643) (-6.9651, -15.8695) (-6.9658, -15.8748) (-6.9665, -15.8802) (-6.9672, -15.8856) (-6.9679, -15.8911) (-6.9686, -15.8966) (-6.9693, -15.9023) (-6.97, -15.908) (-6.9707, -15.9137) (-6.9714, -15.9196) (-6.9721, -15.9255) (-6.9728, -15.9314) (-6.9735, -15.9374) (-6.9742, -15.9435) (-6.9749, -15.9497) (-6.9756, -15.9559) (-6.9763, -15.9622) (-6.9769, -15.9685) (-6.9776, -15.9749) (-6.9783, -15.9814) (-6.9789, -15.9879) (-6.9796, -15.9945) (-6.9803, -16.0011) (-6.9809, -16.0078) (-6.9816, -16.0146) (-6.9822, -16.0214) (-6.9828, -16.0283) (-6.9835, -16.0353) (-6.9841, -16.0423) (-6.9847, -16.0493) (-6.9853, -16.0564) (-6.9859, -16.0636) (-6.9865, -16.0709) (-6.9871, -16.0781) (-6.9877, -16.0855) (-6.9882, -16.0929) (-6.9888, -16.1004) (-6.9894, -16.1079) (-6.9899, -16.1154) (-6.9905, -16.1231) (-6.991, -16.1307) (-6.9915, -16.1385) (-6.9921, -16.1463) (-6.9926, -16.1541) (-6.9931, -16.162) (-6.9936, -16.17) (-6.994, -16.178) (-6.9945, -16.186) (-6.995, -16.1941) (-6.9954, -16.2023) (-6.9959, -16.2105) (-6.9963, -16.2187) (-6.9968, -16.227) (-6.9972, -16.2354) (-6.9976, -16.2438) (-6.998, -16.2523) (-6.9984, -16.2608) (-6.9987, -16.2694) (-6.9991, -16.278) (-6.9995, -16.2866) (-6.9998, -16.2953) (-7.0001, -16.3041) (-7.0005, -16.3129) (-7.0008, -16.3218) (-7.0011, -16.3307) (-7.0014, -16.3396) (-7.0016, -16.3486) (-7.0019, -16.3577) (-7.0021, -16.3668) (-7.0024, -16.3759) (-7.0026, -16.3851) (-7.0028, -16.3943) (-7.003, -16.4036) (-7.0032, -16.4129) (-7.0034, -16.4223) (-7.0036, -16.4317) (-7.0037, -16.4412) (-7.0038, -16.4507) (-7.004, -16.4602) (-7.0041, -16.4698) (-7.0042, -16.4795) (-7.0043, -16.4892) (-7.0043, -16.4989) (-7.0044, -16.5087) (-7.0044, -16.5185) (-7.0045, -16.5284) (-7.0045, -16.5383) (-7.0045, -16.5482) (-7.0045, -16.5582) (-7.0044, -16.5682) (-7.0044, -16.5783) (-7.0043, -16.5884) (-7.0043, -16.5986) (-7.0042, -16.6088) (-7.0041, -16.619) (-7.004, -16.6293) (-7.0038, -16.6396) (-7.0037, -16.65) (-7.0035, -16.6604) (-7.0034, -16.6708) (-7.0032, -16.6813) (-7.003, -16.6919) (-7.0028, -16.7024) (-7.0025, -16.713) (-7.0023, -16.7237) (-7.002, -16.7344) (-7.0017, -16.7451) (-7.0014, -16.7559) (-7.0011, -16.7667) (-7.0008, -16.7775) (-7.0004, -16.7884) (-7.0001, -16.7993) (-6.9997, -16.8103) (-6.9993, -16.8213) (-6.9989, -16.8323) (-6.9984, -16.8434) (-6.998, -16.8545) (-6.9975, -16.8657) (-6.997, -16.8768) (-6.9965, -16.8881) (-6.996, -16.8993) (-6.9955, -16.9106) (-6.995, -16.922) (-6.9944, -16.9333) (-6.9938, -16.9447) (-6.9932, -16.9562) (-6.9926, -16.9677) (-6.992, -16.9792) (-6.9913, -16.9907) (-6.9906, -17.0023) (-6.99, -17.014) (-6.9892, -17.0256) (-6.9885, -17.0373) (-6.9878, -17.049) (-6.987, -17.0608) (-6.9863, -17.0726) (-6.9855, -17.0844) (-6.9846, -17.0963) (-6.9838, -17.1082) (-6.983, -17.1201) (-6.9821, -17.1321) (-6.9812, -17.1441) (-6.9803, -17.1562) (-6.9794, -17.1682) (-6.9784, -17.1803) (-6.9775, -17.1925) (-6.9765, -17.2047) (-6.9755, -17.2169) (-6.9745, -17.2291) (-6.9735, -17.2414) (-6.9724, -17.2537) (-6.9713, -17.266) (-6.9702, -17.2784) (-6.9691, -17.2908) (-6.968, -17.3032) (-6.9669, -17.3157) (-6.9657, -17.3282) (-6.9645, -17.3407) (-6.9633, -17.3533) (-6.9621, -17.3659) (-6.9608, -17.3785) (-6.9596, -17.3912) (-6.9583, -17.4039) (-6.957, -17.4166) (-6.9556, -17.4293) (-6.9543, -17.4421) (-6.9529, -17.4549) (-6.9516, -17.4678) (-6.9501, -17.4806) (-6.9487, -17.4935) (-6.9473, -17.5065) (-6.9458, -17.5194) (-6.9443, -17.5324) (-6.9428, -17.5455) (-6.9413, -17.5585) (-6.9398, -17.5716) (-6.9382, -17.5847) (-6.9366, -17.5979) (-6.935, -17.611) (-6.9334, -17.6242) (-6.9317, -17.6375) (-6.9301, -17.6507) (-6.9284, -17.664) (-6.9267, -17.6773) (-6.925, -17.6907) (-6.9236, -17.7014) (-6.9225, -17.7094) (-6.9218, -17.7148) (-6.9214, -17.7174) knots 0 0 0 0 0 0 0.00416667 0.00833333 0.0125 0.01666667 0.02083333 0.025 0.02916667 0.03333333 0.0375 0.04166667 0.04583333 0.05 0.05416667 0.05833333 0.0625 0.06666667 0.07083333 0.075 0.07916667 0.08333333 0.0875 0.09166667 0.09583333 0.1 0.10416667 0.10833333 0.1125 0.11666667 0.12083333 0.125 0.12916667 0.13333333 0.1375 0.14166667 0.14583333 0.15 0.15416667 0.15833333 0.1625 0.16666667 0.17083333 0.175 0.17916667 0.18333333 0.1875 0.19166667 0.19583333 0.2 0.20416667 0.20833333 0.2125 0.21666667 0.22083333 0.225 0.22916667 0.23333333 0.2375 0.24166667 0.24583333 0.25 0.25416667 0.25833333 0.2625 0.26666667 0.27083333 0.275 0.27916667 0.28333333 0.2875 0.29166667 0.29583333 0.3 0.30416667 0.30833333 0.3125 0.31666667 0.32083333 0.325 0.32916667 0.33333333 0.3375 0.34166667 0.34583333 0.35 0.35416667 0.35833333 0.3625 0.36666667 0.37083333 0.375 0.37916667 0.38333333 0.3875 0.39166667 0.39583333 0.4 0.40416667 0.40833333 0.4125 0.41666667 0.42083333 0.425 0.42916667 0.43333333 0.4375 0.44166667 0.44583333 0.45 0.45416667 0.45833333 0.4625 0.46666667 0.47083333 0.475 0.47916667 0.48333333 0.4875 0.49166667 0.49583333 0.5 0.50416667 0.50833333 0.5125 0.51666667 0.52083333 0.525 0.52916667 0.53333333 0.5375 0.54166667 0.54583333 0.55 0.55416667 0.55833333 0.5625 0.56666667 0.57083333 0.575 0.57916667 0.58333333 0.5875 0.59166667 0.59583333 0.6 0.60416667 0.60833333 0.6125 0.61666667 0.62083333 0.625 0.62916667 0.63333333 0.6375 0.64166667 0.64583333 0.65 0.65416667 0.65833333 0.6625 0.66666667 0.67083333 0.675 0.67916667 0.68333333 0.6875 0.69166667 0.69583333 0.7 0.70416667 0.70833333 0.7125 0.71666667 0.72083333 0.725 0.72916667 0.73333333 0.7375 0.74166667 0.74583333 0.75 0.75416667 0.75833333 0.7625 0.76666667 0.77083333 0.775 0.77916667 0.78333333 0.7875 0.79166667 0.79583333 0.8 0.80416667 0.80833333 0.8125 0.81666667 0.82083333 0.825 0.82916667 0.83333333 0.8375 0.84166667 0.84583333 0.85 0.85416667 0.85833333 0.8625 0.86666667 0.87083333 0.875 0.87916667 0.88333333 0.8875 0.89166667 0.89583333 0.9 0.90416667 0.90833333 0.9125 0.91666667 0.92083333 0.925 0.92916667 0.93333333 0.9375 0.94166667 0.94583333 0.95 0.95416667 0.95833333 0.9625 0.96666667 0.97083333 0.975 0.97916667 0.98333333 0.9875 0.99166667 0.99583333 1 1 1 1 1 1
  line L206 (25.6019, -1.2175) -> (25.6012, -1.2171)
  arc A104 (15.1575, -11.9297) -> (16.1526, -11.2836) centre (0, 12.5) ccw